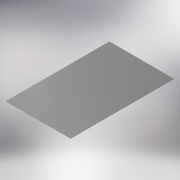
# Autodesk Inventor part: steel-baseplate-400x250
Saved by Autodesk Inventor 2016 (Build 200138000, 138)
## iProperties
Created: 2015-05-19
Part Number: steel-baseplate-400x250
Material: Steel, Mild
Document SubType Name: Modeling
Designer: as
Mass: 785 g
Surface Area: 2013 cm^2
Volume: 100 cm^3
Density: 7.85 g/cm^3
Appearance: Semi-Polished
Author: as
Autodesk Inventor part; units mm, degrees
ref_plane "YZ Plane" through (0, 0, 0) normal (1, 0, 0) x (0, 1, 0)
ref_plane "XZ Plane" through (0, 0, 0) normal (0, 1, 0) x (-1, 0, 0)
ref_plane "XY Plane" through (0, 0, 0) normal (0, 0, 1) x (1, 0, 0)
sketch "Sketch1" plane through (0, 0, 0) normal (0, 0, 1) x (1, 0, 0)
  line L0 (0, 0) -> (-250, 0)
  line L1 (-250, 0) -> (-250, 400)
  line L2 (-250, 400) -> (0, 400)
  line L3 (0, 400) -> (0, 0)
  dimension "d0" = 250
  dimension "d1" = 400
  constraints: 8 end point, 2 parallel, 1 horizontal, 1 perpendicular
  measures "d0" distance of L1.end L2.end
  measures "d1" distance of L0.end L1.end
extrude "Extrusion1" add sketch "Sketch1" along normal blind 1
body "Solid1"
